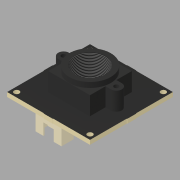
# Autodesk Inventor part: Spinel USB Camera 01 trimmed
Saved by Autodesk Inventor 2019 (Build 230136000, 136)
## iProperties
Created: 2019-03-04
Part Number: Spinel USB Camera 01 trimmed
Material: Generic
Document SubType Name: Modeling
Designer: Ben
Density: 1 g/cm^3
Appearance: Default
Author: Ben
Autodesk Inventor part; units mm, degrees
ref_plane "YZ Plane" through (0, 0, 0) normal (1, 0, 0) x (0, 1, 0)
ref_plane "XZ Plane" through (0, 0, 0) normal (0, 1, 0) x (-1, 0, 0)
ref_plane "XY Plane" through (0, 0, 0) normal (0, 0, 1) x (1, 0, 0)
sketch "Sketch1" plane through (0, 0, 0) normal (0, 1, 0) x (-1, 0, 0)
  line L0 (-19, 19) -> (19, 19)
  line L1 (19, 19) -> (19, -19)
  line L2 (19, -19) -> (-19, -19)
  line L3 (-19, -19) -> (-19, 19)
  line L4 (-19, 19) -> (19, -19) construction
  line L5 (19, 19) -> (-19, -19) construction
  line L6 (-17, -17) -> (17, -17)
  line L7 (17, -17) -> (17, 17)
  line L8 (17, 17) -> (-17, 17)
  line L9 (-17, 17) -> (-17, -17)
  line L10 (16, -16) -> (-16, -16)
  line L11 (-16, -16) -> (-16, 16)
  line L12 (-16, 16) -> (16, 16)
  line L13 (16, 16) -> (16, -16)
  circle A0 centre (17, -17) radius 1
  circle A1 centre (-17, -17) radius 1
  circle A2 centre (-17, 17) radius 1
  circle A3 centre (17, 17) radius 1
  line L14 (16, 16) -> (14.15, 16) construction
  line L15 (14.15, 16) -> (14.15, 14.15) construction
  line L16 (14.15, 14.15) -> (16, 14.15) construction
  line L17 (16, 14.15) -> (16, 16) construction
  circle A4 centre (14.15, 14.15) radius 1
  circle A5 centre (-14.15, 14.15) radius 1
  circle A6 centre (-14.15, -14.15) radius 1
  circle A7 centre (14.15, -14.15) radius 1
  line L18 (0, 16) -> (0, 17) construction
  line L19 (-1.5, 17) -> (1.5, 17)
  line L20 (1.5, 17) -> (1.5, 16)
  line L21 (1.5, 16) -> (-1.5, 16)
  line L22 (-1.5, 16) -> (-1.5, 17)
  line L23 (-1.5, 17) -> (1.5, 16) construction
  line L24 (1.5, 17) -> (-1.5, 16) construction
  line L25 (-17, 1.5) -> (-16, 1.5)
  line L26 (-16, 0) -> (-17, 0) construction
  line L27 (-16, 1.5) -> (-16, -1.5)
  line L28 (-16, -1.5) -> (-17, -1.5)
  line L29 (-17, -1.5) -> (-17, 1.5)
  line L30 (-17, 1.5) -> (-16, -1.5) construction
  line L31 (-17, -1.5) -> (-16, 1.5) construction
  line L32 (-1.5, -17) -> (-1.5, -16)
  line L33 (0, -16) -> (0, -17) construction
  line L34 (-1.5, -16) -> (1.5, -16)
  line L35 (1.5, -16) -> (1.5, -17)
  line L36 (1.5, -17) -> (-1.5, -17)
  line L37 (-1.5, -17) -> (1.5, -16) construction
  line L38 (1.5, -17) -> (-1.5, -16) construction
  line L39 (17, -1.5) -> (16, -1.5)
  line L40 (16, 0) -> (17, 0) construction
  line L41 (16, -1.5) -> (16, 1.5)
  line L42 (16, 1.5) -> (17, 1.5)
  line L43 (17, 1.5) -> (17, -1.5)
  line L44 (17, -1.5) -> (16, 1.5) construction
  line L45 (17, 1.5) -> (16, -1.5) construction
  point P0 (0, 0)
  point P1 (0, 16.5)
  point P2 (-16.5, 0)
  point P3 (0, -16.5)
  point P4 (16.5, 0)
  dimension "d49" = 2
  dimension "d0" = 38
  dimension "d1" = 38
  dimension "d2" = 2
  dimension "d3" = 1
  dimension "d4" = 2
  dimension "d5" = 2
  dimension "d6" = 2
  dimension "d7" = 2
  dimension "d8" = 1.85
  dimension "d9" = 1.85
  dimension "d10" = 2
  dimension "d13" = 360
  dimension "d15" = 3
  dimension "d18" = 360
  constraints: 92 end point, 13 midpoint, 10 parallel, 8 centre point, 5 coincident, 5 perpendicular, 3 horizontal, 1 point on line, 72 other
  measures "d0" distance of L1.end L2.end
  measures "d1" distance of L0.end L1.end
  measures "d2" distance between parallel lines of L2 L6
  measures "d3" distance between parallel lines of L6 L10
  measures "d4" diameter of A0
  measures "d5" diameter of A1
  measures "d6" diameter of A2
  measures "d7" diameter of A3
  measures "d8" distance of L16.end L15.end
  measures "d9" distance of L15.end L14.end
  measures "d10" diameter of A4
  measures "d15" distance of L20.end L21.end
extrude "Extrusion1" add sketch "Sketch1" along normal blind 1.65 contours L0 L1 L2 L3 | L32 L10 L35 L6 | L9 L25 L11 L28 | L10 L11 L12 L13 | L39 L13 L42 L7 | L8 L20 L12 L22
fillet "Fillet1" radius 0.5 16 edges at (-17, 0.825, 1.5) (-16, 0.825, 1.5) (-17, 0.825, -1.5) (-16, 0.825, -1.5) (-1.5, 0.825, -16) (1.5, 0.825, -16) (1.5, 0.825, -17) (-1.5, 0.825, -17) (16, 0.825, -1.5) (17, 0.825, -1.5) (17, 0.825, 1.5) (16, 0.825, 1.5) (1.5, 0.825, 16) (-1.5, 0.825, 16) (-1.5, 0.825, 17) (1.5, 0.825, 17)
sketch "Sketch2" plane through (0, 1.65, 0) normal (0, 1, 0) x (1, 0, 0)
  line L0 (8.075, -8.075) -> (-8.075, -8.075)
  line L1 (-8.075, -8.075) -> (-8.075, 8.075)
  line L2 (-8.075, 8.075) -> (8.075, 8.075)
  line L3 (8.075, 8.075) -> (8.075, -8.075)
  line L4 (8.075, -8.075) -> (-8.075, 8.075) construction
  line L5 (-8.075, -8.075) -> (8.075, 8.075) construction
  line L6 (-8.075, 0) -> (-10.175, 0) construction
  line L7 (8.075, 0) -> (10.175, 0) construction
  line L8 (-8.075, -2.1) -> (-10.175, -2.1)
  line L9 (-12.275, 0) -> (-12.275, 0)
  line L10 (-10.175, 2.1) -> (-8.075, 2.1)
  line L11 (-8.075, 2.1) -> (-8.075, -2.1)
  line L12 (-8.075, -2.1) -> (-12.275, 2.1) construction
  line L13 (-12.275, -2.1) -> (-8.075, 2.1) construction
  line L14 (8.075, -2.1) -> (10.175, -2.1)
  line L15 (12.275, 0) -> (12.275, 0)
  line L16 (10.175, 2.1) -> (8.075, 2.1)
  line L17 (8.075, 2.1) -> (8.075, -2.1)
  line L18 (8.075, -2.1) -> (12.275, 2.1) construction
  line L19 (12.275, -2.1) -> (8.075, 2.1) construction
  arc A0 (-10.175, 2.1) -> (-12.275, 0) centre (-10.175, 0) ccw
  arc A1 (-12.275, 0) -> (-10.175, -2.1) centre (-10.175, 0) ccw
  arc A2 (10.175, -2.1) -> (12.275, 0) centre (10.175, 0) ccw
  arc A3 (12.275, 0) -> (10.175, 2.1) centre (10.175, 0) ccw
  circle A4 centre (-10.175, 0) radius 0.875
  circle A5 centre (10.175, 0) radius 0.875
  point P0 (0, 0)
  dimension "d23" = 16.15
  dimension "d24" = 16.15
  dimension "d25" = 2.1
  dimension "d26" = 2.1
  dimension "d27" = 4.2
  dimension "d28" = 4.2
  dimension "d29" = 4.2
  dimension "d30" = 4.2
  dimension "d31" = 2.1
  dimension "d34" = 1.75
  dimension "d35" = 1.75
  constraints: 40 end point, 8 midpoint, 8 point on circle, 8 point on line, 8 tangent, 6 centre point, 6 parallel, 5 horizontal, 3 equal radius, 3 perpendicular, 2 coincident
  measures "d23" distance of L1.end L2.end
  measures "d24" distance of L0.end L1.end
  measures "d25" distance of L6.start L6.end
  measures "d26" distance of L7.start L7.end
  measures "d27" distance of L12.end L10.end
  measures "d28" distance of L13.start L12.end
  measures "d29" distance of L16.end L18.end
  measures "d30" distance of L18.end L19.start
  measures "d31" radius of A0
  measures "d34" diameter of A4
  measures "d35" diameter of A5
extrude "Extrusion2" add sketch "Sketch2" along normal blind 7 separate body
sketch "Sketch3" plane through (0, 0, 0) normal (0, -1, 0) x (1, 0, 0)
  line L0 (5, 11.3) -> (-5, 11.3)
  line L1 (-5, 11.3) -> (-5, 16)
  line L2 (-5, 16) -> (5, 16)
  line L3 (5, 16) -> (5, 11.3)
  line L4 (2, 16) -> (16, 16) projected
  point P0 (0, 0)
  dimension "d36" = 10
  dimension "d37" = 4.7
  dimension "d38" = 5
  constraints: 8 end point, 2 parallel, 1 collinear, 1 horizontal, 1 perpendicular
  measures "d36" distance of L1.end L2.end
  measures "d37" distance of L0.end L1.end
  measures "d38" distance from line of point (0, 0) L3
extrude "Extrusion3" add sketch "Sketch3" along normal blind 6 separate body
sketch "Sketch4" plane through (0, -6, 0) normal (0, -1, 0) x (1, 0, 0)
  line L0 (-5, 11.3) -> (5, 11.3) projected
  line L1 (5, 11.3) -> (5, 16) projected
  line L2 (5, 16) -> (-5, 16) projected
  line L3 (-5, 16) -> (-5, 11.3) projected
  line L4 (4.5, 11.8) -> (-4.5, 11.8)
  line L5 (-4.5, 11.8) -> (-4.5, 15.5)
  line L6 (-4.5, 15.5) -> (4.5, 15.5)
  line L7 (4.5, 15.5) -> (4.5, 11.8)
  line L8 (5, 16) -> (-5, 16) projected
  line L9 (2, 15.5) -> (-2, 15.5)
  line L10 (-2, 15.5) -> (-2, 16)
  line L11 (-2, 16) -> (2, 16)
  line L12 (2, 16) -> (2, 15.5)
  point P0 (0, 0)
  dimension "d41" = 0.5
  dimension "d42" = 4
  dimension "d43" = 2
  constraints: 16 end point, 2 parallel, 2 point on line, 1 horizontal, 1 perpendicular, 3 other
  measures "d41" distance between parallel lines of L0 L4
  measures "d42" distance of L10.end L11.end
  measures "d43" distance from line of point (0, 0) L12
extrude "Extrusion4" cut sketch "Sketch4" against normal blind 4.5 contours L2 L12 L6 L10 | L6 L7 L4 L5 bodies 3
sketch "Sketch5" plane through (0, 8.65, 0) normal (0, 1, 0) x (1, 0, 0)
  circle A0 centre (0, 0) radius 8
  dimension "d46" = 16
  constraints: 1 centre point, 1 coincident
  measures "d46" diameter of A0
extrude "Extrusion5" add sketch "Sketch5" along normal blind 2 bodies 2
sketch "Sketch6" plane through (0, 10.65, 0) normal (0, 1, 0) x (1, 0, 0)
  circle A0 centre (0, 0) radius 8 construction
  circle A1 centre (0, 0) radius 6
  dimension "d49" = 2
  constraints: 1 centre point
  measures "d49" radial gap between concentric circles of A0 A1
extrude "Extrusion6" cut sketch "Sketch6" against normal up to surface (9 mm away) bodies 2
thread "Thread1" size "M12x0.5" class "6H" standard "ANSI Metric M Profile" full length
sketch "Sketch7" plane through (0, 0, 0) normal (0, -1, 0) x (1, 0, 0)
  line L0 (16, 16) -> (-16, 16) construction
  line L1 (-16, 16) -> (-16, -16) construction
  line L2 (-16, -16) -> (16, -16) construction
  line L3 (16, -16) -> (16, 16) construction
  line L4 (16.15, 16.15) -> (-16.15, 16.15)
  line L5 (-16.15, 16.15) -> (-16.15, -16.15)
  line L6 (-16.15, -16.15) -> (16.15, -16.15)
  line L7 (16.15, -16.15) -> (16.15, 16.15)
  line L8 (21.15, 21.15) -> (-21.15, 21.15)
  line L9 (-21.15, 21.15) -> (-21.15, -21.15)
  line L10 (-21.15, -21.15) -> (21.15, -21.15)
  line L11 (21.15, -21.15) -> (21.15, 21.15)
  point P0 (0, 0)
  dimension "d54" = 0.15
  dimension "d55" = 5
  constraints: 24 end point, 6 parallel, 3 perpendicular, 1 horizontal, 6 other
  measures "d54" distance between parallel lines of L3 L7
  measures "d55" distance between parallel lines of L7 L11
extrude "Extrusion7" cut sketch "Sketch7" against normal up to surface (1.65 mm away) bodies 1
equation "\"d38\" = 0.5 * d36"
body "Solid1"
body "Solid2"
body "Solid3"
